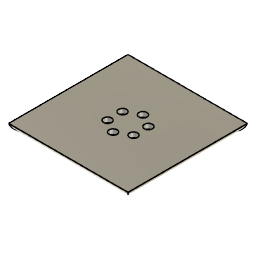
Base v1 (Autodesk Fusion 360 design; units mm, degrees)
Autodesk Fusion 360 part; units mm, degrees
sketch "Sketch1" plane through (0, 0, 0) normal (0, 0, 1) x (1, 0, 0)
  line L0 (60, -60) -> (-60, -60)
  line L1 (-60, -60) -> (-60, 60)
  line L2 (-60, 60) -> (60, 60)
  line L3 (60, 60) -> (60, -60)
  line L4 (60, -60) -> (-60, 60) construction
  line L5 (-60, -60) -> (60, 60) construction
  circle A0 centre (0, 0) radius 15
  circle A1 centre (0, 15) radius 2.15
  circle A2 centre (-12.9904, 7.5) radius 2.15
  circle A3 centre (-12.9904, -7.5) radius 2.15
  circle A4 centre (0, -15) radius 2.15
  circle A5 centre (12.9904, -7.5) radius 2.15
  circle A6 centre (12.9904, 7.5) radius 2.15
  dimension "d1" = 120
  dimension "d2" = 120
  dimension "d3" = 30
  dimension "d4" = 4.3
  dimension "d6" = 360
  constraint horizontal L0
  constraint perpendicular L0 L1
  constraint parallel L0 L2
  constraint parallel L1 L3
  constraint coincident L4 A0.centre
  constraint coincident L5 A0.centre
  constraint coincident A0.centre origin
  constraint coincident A0 A1.centre
  measures "d1" distance of L1.end L2.end
  measures "d2" distance of L0.end L1.end
  measures "d3" diameter of A0
  measures "d4" diameter of A1
extrude "Extrude1" add sketch "Sketch1" along normal blind 8 contours L0 L1 L2 L3 | A0 A1 A2 A3 A4 A5 A6
sketch "Sketch2" plane through (0, 0, 8) normal (0, 0, 1) x (-1, 0, 0)
  circle A0 centre (12.9904, 7.5) radius 2.15
  circle A1 centre (0, 15) radius 2.15
  circle A2 centre (-12.9904, 7.5) radius 2.15
  circle A3 centre (-12.9904, -7.5) radius 2.15
  circle A4 centre (0, -15) radius 2.15
  circle A5 centre (12.9904, -7.5) radius 2.15
  line L0 (-60, -60) -> (60, -60)
  line L1 (60, -60) -> (60, 60)
  line L2 (60, 60) -> (-60, 60)
  line L3 (-60, 60) -> (-60, -60)
  circle A6 centre (0, -15) radius 4
  circle A7 centre (-12.9904, -7.5) radius 4
  circle A8 centre (-12.9904, 7.5) radius 4
  circle A9 centre (0, 15) radius 4
  circle A10 centre (12.9904, 7.5) radius 4
  circle A11 centre (12.9904, -7.5) radius 4
  dimension "d9" = 8
  dimension "d10" = 8
  dimension "d11" = 8
  dimension "d12" = 8
  dimension "d13" = 8
  dimension "d14" = 8
  constraint concentric A4 A6
  constraint concentric A3 A7
  constraint concentric A2 A8
  constraint concentric A1 A9
  constraint concentric A0 A10
  constraint concentric A5 A11
  measures "d9" diameter of A6
  measures "d10" diameter of A7
  measures "d11" diameter of A8
  measures "d12" diameter of A9
  measures "d13" diameter of A10
  measures "d14" diameter of A11
extrude "Extrude2" cut sketch "Sketch2" against normal blind 5 contours A6 | A7 | A8 | A9 | A10 | A11
fillet "Fillet1" radius 10 4 edges at (0, -60, 0) (-60, 0, 0) (60, 0, 0) (0, 60, 0)
